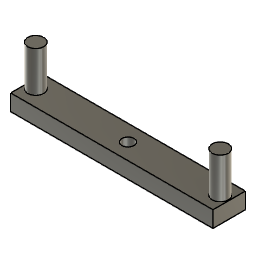
MIttenfinder-L_v1 (Autodesk Fusion 360 design; units mm, degrees)
Autodesk Fusion 360 part; units mm, degrees
sketch "Skizze1" plane through (0, 0, 0) normal (0, 0, 1) x (1, 0, 0)
  line L0 (0, 0) -> (125, 0)
  line L1 (125, 0) -> (125, 20)
  line L2 (125, 20) -> (0, 20)
  line L3 (0, 20) -> (0, 0)
  dimension "d1" = 125
  dimension "d2" = 20
  constraint horizontal L0
  constraint vertical L1
  constraint horizontal L2
  constraint vertical L3
  constraint coincident L0.start L3.end
  measures "d1" distance of L0.start L0.end
  measures "d2" distance of L0.start L2.end
extrude "Extrusion1" add sketch "Skizze1" along normal blind 10
sketch "Skizze2" plane through (0, 0, 10) normal (0, 0, 1) x (-1, 0, 0)
  line L0 (0, -20) -> (0, 0)
  line L1 (0, 0) -> (-125, 0)
  line L2 (-125, 0) -> (-125, -20)
  line L3 (-125, -20) -> (0, -20)
  circle A0 centre (-62.5, -10) radius 3.75
  dimension "d5" = 7.5
  measures "d5" diameter of A0
extrude "Extrusion2" cut sketch "Skizze2" against normal blind 10 contours A0
sketch "Skizze3" plane through (0, 0, 10) normal (0, 0, 1) x (-1, 0, 0)
  circle A0 centre (-62.5, -10) radius 3.75
  line L0 (0, -20) -> (0, 0)
  line L1 (0, 0) -> (-125, 0)
  line L2 (-125, 0) -> (-125, -20)
  line L3 (-125, -20) -> (0, -20)
  line L4 (0, -10, -5) -> (-125, -10, 0)
  line L5 (0, -10, -5) -> (-5.5, -10, -5)
  line L6 (-125, -10) -> (-119.5, -10)
  circle A1 centre (-5.5026, -10) radius 5
  circle A2 centre (-119.5, -10) radius 5
  dimension "d8" = 5.5
  dimension "d9" = 5.5
  dimension "d10" = 10
  dimension "d13" = 10
  constraint midpoint L2 L6.start
  constraint perpendicular L2 L6
  constraint coincident L6.end A2.centre
  measures "d9" distance of L6.start L6.end
  measures "d10" diameter of A1
  measures "d13" diameter of A2
extrude "Extrusion4" add sketch "Skizze3" along normal blind 25 contours A1 | A2
extrude "Extrusion3" add sketch "Skizze3" along normal blind 10 contours A1
sketch "Skizze4" plane through (0, 0, 10) normal (0, 0, 1) x (1, 0, 0)
  circle A0 centre (62.5, 10) radius 3.8
  point P0 (62.5, 10)
  dimension "d16" = 7.6
  constraint coincident P0 A0.centre
  measures "d16" diameter of A0
extrude "Extrusion5" cut sketch "Skizze4" against normal blind 20
sketch "Skizze5" plane through (0, 0, 10) normal (0, 0, 1) x (1, 0, 0)
